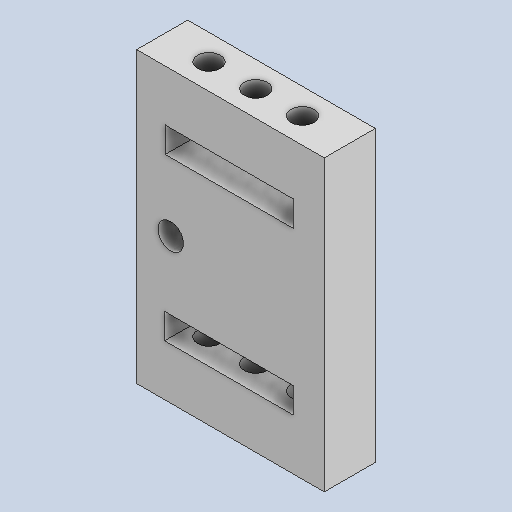
# Autodesk Inventor part: _adle_adt_2
Saved by Autodesk Inventor 2024.3 (Build 283343000, 343)
## iProperties
Created: 2024-09-05
Part Number: _adle_adt_2
Material: 일반
Document SubType Name: Modeling
Designer: gretc
Density: 1 g/cm^3
Appearance: 기본값
Author: gretc
Autodesk Inventor part; units mm, degrees
ref_plane "YZ Plane" through (0, 0, 0) normal (1, 0, 0) x (0, 1, 0)
ref_plane "XZ Plane" through (0, 0, 0) normal (0, 1, 0) x (-1, 0, 0)
ref_plane "XY Plane" through (0, 0, 0) normal (0, 0, 1) x (1, 0, 0)
sketch "스케치1" plane through (0, 0, 0) normal (0, 0, 1) x (1, 0, 0)
  line L0 (28.5, 0) -> (46.5, 0) projected
  line L1 (46.5, 0) -> (46.5, -1.5) projected
  line L2 (50.5, -1.5) -> (46.5, -1.5) projected
  line L3 (50.5, 0) -> (50.5, -1.5) projected
  line L4 (50.5, 0) -> (53.1, 0) projected
  line L5 (53.1, 0) -> (53.1, 2) projected
  line L6 (0, 2) -> (53.1, 2) projected
  line L7 (0, 0) -> (0, 2) projected
  line L8 (0, 0) -> (2.5, 0) projected
  line L9 (2.5, 0) -> (2.5, -1.5) projected
  line L10 (6.5, -1.5) -> (2.5, -1.5) projected
  line L11 (6.5, 0) -> (6.5, -1.5) projected
  line L12 (6.5, 0) -> (24.5, 0) projected
  line L13 (24.5, 0) -> (24.5, -1.5) projected
  line L14 (28.5, -1.5) -> (24.5, -1.5) projected
  line L15 (28.5, 0) -> (28.5, -1.5) projected
  line L16 (8.475, -27.5) -> (6.975, -27.5) projected
  line L17 (6.975, -27.5) -> (6.975, -29.5) projected
  line L18 (6.975, -29.5) -> (2.025, -29.5) projected
  line L19 (2.025, -27.5) -> (2.025, -29.5) projected
  line L20 (2.025, -27.5) -> (0.525, -27.5) projected
  line L21 (0.525, -27.5) -> (0.525, -30) projected
  line L22 (0, -30) -> (0.525, -30) projected
  line L23 (0, -30) -> (0, -32) projected
  line L24 (0, -32) -> (53.1, -32) projected
  line L25 (53.1, -30) -> (53.1, -32) projected
  line L26 (52.475, -30) -> (53.1, -30) projected
  line L27 (52.475, -30) -> (52.475, -27.5) projected
  line L28 (52.475, -27.5) -> (50.975, -27.5) projected
  line L29 (50.975, -27.5) -> (50.975, -29.5) projected
  line L30 (50.975, -29.5) -> (46.025, -29.5) projected
  line L31 (46.025, -27.5) -> (46.025, -29.5) projected
  line L32 (46.025, -27.5) -> (44.525, -27.5) projected
  line L33 (44.525, -27.5) -> (44.525, -30) projected
  line L34 (30.475, -30) -> (44.525, -30) projected
  line L35 (30.475, -30) -> (30.475, -27.5) projected
  line L36 (30.475, -27.5) -> (28.975, -27.5) projected
  line L37 (28.975, -27.5) -> (28.975, -29.5) projected
  line L38 (28.975, -29.5) -> (24.025, -29.5) projected
  line L39 (24.025, -27.5) -> (24.025, -29.5) projected
  line L40 (24.025, -27.5) -> (22.525, -27.5) projected
  line L41 (22.525, -27.5) -> (22.525, -30) projected
  line L42 (8.475, -30) -> (22.525, -30) projected
  line L43 (8.475, -30) -> (8.475, -27.5) projected
  line L44 (48.1766, 5.1) -> (3.9234, 5.1) projected
  line L45 (29.3, 2) -> (29.3, 8)
  line L46 (3.15, 8) -> (3.15, 2)
  line L47 (1.7, -38) -> (1.7, -32)
  line L48 (29.3, -38) -> (29.3, -32)
  line L49 (15.5, 2) -> (15.5, -15)
  circle A0 centre (8.5, -15) radius 1.5 projected
  line L50 (26.55, 2) -> (26.55, -32)
  line L51 (4.5, 2) -> (4.5, -32)
  dimension "d0" = 17
  constraints: 14 end point, 7 vertical, 3 point on line, 2 midpoint, 1 coincident, 8 other
  measures "d0" distance of L49.start L49.end
extrude "돌출1" add sketch "스케치1" along normal blind 6 contours L50 L38 L39 L40 L41 L42 L43 L16 L17 L18 L51 L10 L11 L12 L13 L14 | L14 L13 L12 L49 L6 L50 | L50 L24 L51 L18 L17 L16 L43 L42 L41 L40 L39 L38 | L49 L12 L11 L10 L51 L6
sketch "스케치2" plane through (4.5, 2, 0) normal (0, 1, 0) x (1, 0, 0)
  arc A0 (22, 0) -> (22, 5.6) centre (22, 2.8) ccw projected
  line L0 (22, 5.6) -> (0, 5.6) projected
  arc A1 (0, 5.6) -> (0, 0) centre (0, 2.8) ccw projected
  line L1 (0, 0) -> (0, -6) projected
  line L2 (0, -6) -> (22, -6) projected
  line L3 (22, -6) -> (22, 0) projected
  circle A2 centre (11, -3) radius 1.35 projected
  circle A3 centre (16.5, -3) radius 1.35 projected
  circle A4 centre (0, 2.8) radius 1.35 projected
  circle A5 centre (22, 2.8) radius 1.35 projected
  circle A6 centre (5.5, -3) radius 1.35 projected
  point P0 (-4.5, 0)
extrude "돌출2" cut sketch "스케치2" against normal blind 6 contours A2 | A3 | A6
sketch "스케치3" plane through (4.5, -32, 0) normal (0, -1, 0) x (1, 0, 0)
  arc A0 (22, -5.6) -> (22, 0) centre (22, -2.8) ccw projected
  line L0 (22, 6) -> (22, 0) projected
  line L1 (0, 6) -> (22, 6) projected
  line L2 (0, 0) -> (0, 6) projected
  arc A1 (0, 0) -> (0, -5.6) centre (0, -2.8) ccw projected
  line L3 (22, -5.6) -> (0, -5.6) projected
  circle A2 centre (11, 3) radius 1.35 projected
  circle A3 centre (16.5, 3) radius 1.35 projected
  circle A4 centre (0, -2.8) radius 1.35 projected
  circle A5 centre (22, -2.8) radius 1.35 projected
  circle A6 centre (5.5, 3) radius 1.35 projected
  point P0 (-4.5, 0)
extrude "돌출3" cut sketch "스케치3" against normal blind 6 contours A2 | A3 | A6
sketch "스케치4" plane through (0, 0, 6) normal (0, 0, 1) x (1, 0, 0)
  line L0 (19.65, -4) -> (22.35, -4) projected
  line L1 (14.15, -4) -> (16.85, -4) projected
  line L2 (8.65, -4) -> (11.35, -4) projected
  line L3 (22.35, -26) -> (19.65, -26) projected
  line L4 (16.85, -26) -> (14.15, -26) projected
  line L5 (11.35, -26) -> (8.65, -26) projected
  line L6 (22.883, -4) -> (22.883, -7)
  line L7 (22.883, -7) -> (7.8508, -7)
  line L8 (7.8508, -7) -> (7.8508, -4)
  line L9 (7.8508, -4) -> (22.883, -4)
  line L10 (22.883, -23) -> (22.883, -26)
  line L11 (22.883, -26) -> (7.788, -26)
  line L12 (7.788, -26) -> (7.788, -23)
  line L13 (7.788, -23) -> (22.883, -23)
  line L14 (8.65, -32) -> (8.65, -26) projected
  line L15 (8.65, 2) -> (8.65, -4) projected
  point P0 (0, 0)
  dimension "d7" = 3
  dimension "d8" = 3
  constraints: 16 end point, 4 parallel, 2 perpendicular, 2 vertical
  measures "d7" distance of L6.start L6.end
  measures "d8" distance of L10.end L10.start
extrude "돌출4" cut sketch "스케치4" against normal blind 3
